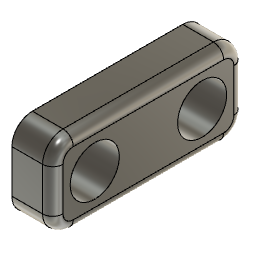
probe_retainer_bracket (Autodesk Fusion 360 design; units mm, degrees)
Autodesk Fusion 360 part; units mm, degrees
sketch "Sketch1" plane through (0, 0, 0) normal (1, 0, 0) x (0, 1, 0) in component "probe_retainer_bracket"
  line L0 (9.35, 4.1) -> (-9.35, 4.1)
  line L1 (-9.35, 4.1) -> (-9.35, -4.1)
  line L2 (-9.35, -4.1) -> (9.35, -4.1)
  line L3 (9.35, -4.1) -> (9.35, 4.1)
  line L4 (9.35, 4.1) -> (-9.35, -4.1) construction
  line L5 (-9.35, 4.1) -> (9.35, -4.1) construction
  circle A0 centre (-5.25, -0.0082) radius 2.4
  line L6 (0, 0) -> (-10.0428, -0.0157) construction
  line L7 (0, 0) -> (0, 6) construction
  circle A1 centre (5.25, -0.0082) radius 2.4
  dimension "d1" = 18.7
  dimension "d2" = 8.2
  dimension "d3" = 4.8
  dimension "d4" = 10.5
  constraint horizontal L0
  constraint perpendicular L0 L1
  constraint parallel L0 L2
  constraint parallel L1 L3
  constraint coincident L4 L6.start
  constraint coincident L5 L6.start
  constraint coincident L6.start L7.start
  constraint coincident A0.centre L6
  constraint perpendicular L0 L7
  constraint symmetric A0 L7 A1
  measures "d1" distance of L1.end L2.end
  measures "d2" distance of L0.end L1.end
  measures "d3" diameter of A0
  measures "d4" distance of A0.centre A1.centre
extrude "Extrude1" add sketch "Sketch1" along normal mid plane 4 in component "probe_retainer_bracket"
fillet "Fillet1" radius 2 4 edges at (0, -9.35, 4.1) (0, 9.35, 4.1) (0, -9.35, -4.1) (0, 9.35, -4.1) in component "probe_retainer_bracket"
fillet "Fillet2" radius 1 8 edges at (2, -8.7642, 3.5142) (2, -9.35, 0) (2, -8.7642, -3.5142) (2, 0, -4.1) (2, 8.7642, -3.5142) (2, 9.35, 0) (2, 8.7642, 3.5142) (2, 0, 4.1) in component "probe_retainer_bracket"
component "probe_retainer_bracket" placed x (1, 0, 0) y (0, 1, 0) z (0, 0, 1) at (0, 0, 0)
